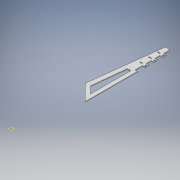
# Autodesk Inventor part: bok
Saved by Autodesk Inventor 2017 (Build 210142000, 142)
## iProperties
Created: 2019-10-27
Part Number: bok
Material: Ogólny
Document SubType Name: Modeling
Designer: patry
Density: 1 g/cm^3
Appearance: Domyślna
Author: patry
Autodesk Inventor part; units mm, degrees
ref_plane "YZ Plane" through (0, 0, 0) normal (1, 0, 0) x (0, 1, 0)
ref_plane "XZ Plane" through (0, 0, 0) normal (0, 1, 0) x (-1, 0, 0)
ref_plane "XY Plane" through (0, 0, 0) normal (0, 0, 1) x (1, 0, 0)
sketch "Szkic1" plane through (0, 0, 0) normal (0, 0, 1) x (1, 0, 0)
  line L0 (176.3308, 486.6406) -> (176.3308, 940.0878) construction
  line L1 (146.3308, 1046.0878) -> (146.3308, 531.0878) construction
  line L2 (246.3308, 494.0715) -> (246.3308, 1046.1041) construction
  line L3 (-96.6896, 915.5533) -> (106.9406, 915.5533) construction
  line L4 (106.9406, 482.7854) -> (106.9406, 1180.5533)
  line L5 (106.9406, 482.7854) -> (-19.1, 609.3854)
  line L6 (50.6014, 1180.5533) -> (-19.1, 609.3854)
  line L7 (19.8894, 612.8224) -> (76.2561, 1146.5389)
  line L8 (76.2561, 1146.5389) -> (76.2561, 556.2056)
  line L9 (43.2451, 833.9694) -> (8.8194, 838.1705) construction
  line L10 (76.2561, 556.2056) -> (54.9566, 535.0002) construction
  line L11 (76.2561, 613.2072) -> (106.9406, 613.2072) construction
  line L12 (76.2561, 556.2056) -> (19.8894, 612.8224)
  line L13 (14.654, 575.0721) -> (120.72, 469.0061) construction
  line L14 (10.3406, 579.3854) -> (14.654, 575.0721) construction
  line L15 (-19.1, 622) -> (-19.1, 0) construction
  line L16 (-8.2, 622) -> (-16.1, 622) construction
  line L17 (-6.6931, 622) -> (-1.5069, 622) construction
  line L18 (-19.1, 622) -> (-16.1, 622) construction
  line L19 (7.9, 622) -> (0, 622) construction
  line L20 (10.9, 621.8118) -> (36.4266, 596.2853) construction
  line L21 (36.4266, 596.2853) -> (142.1601, 489.8877) construction
  line L22 (48.0033, 879.023) -> (76.2561, 879.023)
  line L23 (91.9406, 1180.5533) -> (424.3104, 1180.5533) construction
  line L24 (106.9406, 915.5533) -> (383.3104, 915.5533) construction
  line L25 (91.9406, 1180.5533) -> (50.6014, 1180.5533)
  line L26 (106.9406, 1180.5533) -> (50.6014, 1180.5533)
  point P0 (0, 0)
  dimension "d0" = 30
  dimension "d1" = 100
  constraints: 54 end point, 14 point on line, 6 perpendicular, 4 horizontal, 3 vertical, 1 parallel
  measures "d0" distance between parallel lines of L0 L1
  measures "d1" distance between parallel lines of L1 L2
ref_plane "Płaszczyzna konstrukcyjna1" through (0, 0, 5) normal (0, 0, 1) x (1, 0, 0)
extrude "Wyciągnięcie proste4" add sketch "Szkic1" along normal blind 5 contours L5 L6 L25 L26 L4 | L7 L8 L22
sketch "Szkic3" plane through (0, 0, 0) normal (0, 0, -1) x (-1, 0, 0)
  line L0 (-48.0033, 879.023) -> (-19.8894, 612.8224) projected
  line L1 (-19.8894, 612.8224) -> (-76.2561, 556.2056) projected
  line L2 (-76.2561, 556.2056) -> (-76.2561, 879.023) projected
  line L3 (-76.2561, 879.023) -> (-48.0033, 879.023) projected
  line L4 (-106.9406, 1180.5533) -> (-106.9406, 482.7854) projected
  line L5 (-106.9406, 482.7854) -> (19.1, 609.3854) projected
  line L6 (19.1, 609.3854) -> (-50.6014, 1180.5533) projected
  line L7 (-50.6014, 1180.5533) -> (-106.9406, 1180.5533) construction
  line L8 (-106.9406, 482.7854) -> (-106.9406, 1180.5533) projected
  line L9 (-106.9406, 1060.5533) -> (-86.9406, 1060.5533)
  line L10 (-86.9406, 1060.5533) -> (-86.9406, 1100.5533)
  line L11 (-86.9406, 1100.5533) -> (-106.9406, 1100.5533)
  line L12 (-106.9406, 1100.5533) -> (-106.9406, 1060.5533)
  line L13 (-106.9406, 1130.5533) -> (-86.9406, 1130.5533)
  line L14 (-86.9406, 1130.5533) -> (-86.9406, 1180.5533)
  line L15 (-86.9406, 1180.5533) -> (-106.9406, 1180.5533)
  line L16 (-106.9406, 1180.5533) -> (-106.9406, 1130.5533)
  line L17 (-106.9406, 1030.5533) -> (-86.9406, 1030.5533)
  line L18 (-86.9406, 1030.5533) -> (-86.9406, 990.5533)
  line L19 (-86.9406, 990.5533) -> (-106.9406, 990.5533)
  line L20 (-106.9406, 990.5533) -> (-106.9406, 1030.5533)
  line L21 (-226, 915.5533) -> (53, 915.5533) construction
  line L22 (-86.9406, 990.5533) -> (-106.9406, 990.5533)
  line L23 (-106.9406, 990.5533) -> (-106.9406, 960.5533)
  line L24 (-106.9406, 960.5533) -> (-86.9406, 960.5533)
  line L25 (-86.9406, 960.5533) -> (-106.9406, 960.5533)
  line L26 (-106.9406, 960.5533) -> (-106.9406, 900.5533)
  line L27 (-106.9406, 900.5533) -> (-86.9406, 900.5533)
  line L28 (-86.9406, 900.5533) -> (-86.9406, 960.5533)
  line L29 (-101.9406, 968.0533) -> (-95.9406, 968.0533)
  line L30 (-95.9406, 968.0533) -> (-95.9406, 983.0533)
  line L31 (-95.9406, 983.0533) -> (-101.9406, 983.0533)
  line L32 (-101.9406, 983.0533) -> (-101.9406, 968.0533)
  line L33 (-101.9406, 1038.0533) -> (-95.9406, 1038.0533)
  line L34 (-95.9406, 1038.0533) -> (-95.9406, 1053.0533)
  line L35 (-95.9406, 1053.0533) -> (-101.9406, 1053.0533)
  line L36 (-101.9406, 1053.0533) -> (-101.9406, 1038.0533)
  line L37 (-101.9406, 1108.0533) -> (-95.9406, 1108.0533)
  line L38 (-95.9406, 1108.0533) -> (-95.9406, 1123.0533)
  line L39 (-95.9406, 1123.0533) -> (-101.9406, 1123.0533)
  line L40 (-101.9406, 1123.0533) -> (-101.9406, 1108.0533)
  point P0 (0, 0)
  dimension "d28" = 265
  dimension "d30" = 30
  dimension "d31" = 30
  dimension "d32" = 40
  dimension "d33" = 40
  dimension "d34" = 30
  dimension "d38" = 20
  dimension "d39" = 6
  dimension "d40" = 15
  dimension "d41" = 6
  dimension "d42" = 15
  dimension "d43" = 6
  dimension "d44" = 15
  dimension "d45" = 7.5
  dimension "d46" = 7.5
  dimension "d47" = 7.5
  dimension "d48" = 5
  dimension "d49" = 5
  dimension "d64" = 50
  constraints: 64 end point, 15 parallel, 9 horizontal, 9 point on line, 8 perpendicular, 1 collinear
  measures "d28" distance between parallel lines of L7 L21
  measures "d30" distance between parallel lines of L13 L11
  measures "d31" distance between parallel lines of L17 L9
  measures "d32" distance between parallel lines of L11 L9
  measures "d33" distance between parallel lines of L17 L19
  measures "d34" distance between parallel lines of L19 L24
  measures "d38" distance between parallel lines of L8 L14
  measures "d39" distance of L35.end L34.end
  measures "d40" distance of L34.end L33.end
  measures "d41" distance of L39.end L38.end
  measures "d42" distance of L38.end L37.end
  measures "d43" distance of L30.end L31.end
  measures "d44" distance of L29.end L30.end
  measures "d45" distance between parallel lines of L24 L29
  measures "d46" distance from line of L33.end L17
  measures "d47" distance from line of L37.end L11
  measures "d48" distance between parallel lines of L4 L32
  measures "d49" distance between parallel lines of L4 L36
  measures "d64" distance between parallel lines of L7 L13
extrude "Wyciągnięcie proste5" cut sketch "Szkic3" against normal blind 5 contours L15 L14 L13 L4 | L11 L10 L9 L4 | L17 L18 L19 L4 | L24 L28 L27 L4 | L32 L31 L30 L29 | L36 L35 L34 L33 | L40 L39 L38 L37
fillet "Zaokrąglenie1" radius 2 12 edges at (101.9406, 968.0533, 2.5) (95.9406, 968.0533, 2.5) (95.9406, 983.0533, 2.5) (101.9406, 983.0533, 2.5) (101.9406, 1053.0533, 2.5) (101.9406, 1038.0533, 2.5) (95.9406, 1038.0533, 2.5) (95.9406, 1053.0533, 2.5) (95.9406, 1123.0533, 2.5) (95.9406, 1108.0533, 2.5) (101.9406, 1108.0533, 2.5) (101.9406, 1123.0533, 2.5)
sketch "Szkic4" plane through (0, 0, 5) normal (0, 0, 1) x (1, 0, 0)
  line L0 (19.8894, 612.8224) -> (48.0033, 879.023) projected
  line L1 (48.0033, 879.023) -> (76.2561, 879.023) projected
  line L2 (76.2561, 879.023) -> (76.2561, 556.2056) projected
  line L3 (76.2561, 556.2056) -> (19.8894, 612.8224) projected
  line L4 (95.9406, 1110.0533) -> (95.9406, 1121.0533) projected
  arc A0 (97.9406, 1123.0533) -> (95.9406, 1121.0533) centre (97.9406, 1121.0533) ccw projected
  line L5 (97.9406, 1123.0533) -> (99.9406, 1123.0533) projected
  arc A1 (101.9406, 1121.0533) -> (99.9406, 1123.0533) centre (99.9406, 1121.0533) ccw projected
  line L6 (101.9406, 1121.0533) -> (101.9406, 1110.0533) projected
  arc A2 (99.9406, 1108.0533) -> (101.9406, 1110.0533) centre (99.9406, 1110.0533) ccw projected
  line L7 (99.9406, 1108.0533) -> (97.9406, 1108.0533) projected
  arc A3 (95.9406, 1110.0533) -> (97.9406, 1108.0533) centre (97.9406, 1110.0533) ccw projected
  line L8 (95.9406, 970.0533) -> (95.9406, 981.0533) projected
  arc A4 (97.9406, 983.0533) -> (95.9406, 981.0533) centre (97.9406, 981.0533) ccw projected
  line L9 (97.9406, 983.0533) -> (99.9406, 983.0533) projected
  arc A5 (101.9406, 981.0533) -> (99.9406, 983.0533) centre (99.9406, 981.0533) ccw projected
  line L10 (101.9406, 981.0533) -> (101.9406, 970.0533) projected
  arc A6 (99.9406, 968.0533) -> (101.9406, 970.0533) centre (99.9406, 970.0533) ccw projected
  line L11 (99.9406, 968.0533) -> (97.9406, 968.0533) projected
  arc A7 (95.9406, 970.0533) -> (97.9406, 968.0533) centre (97.9406, 970.0533) ccw projected
  line L12 (95.9406, 1040.0533) -> (95.9406, 1051.0533) projected
  arc A8 (97.9406, 1053.0533) -> (95.9406, 1051.0533) centre (97.9406, 1051.0533) ccw projected
  line L13 (97.9406, 1053.0533) -> (99.9406, 1053.0533) projected
  arc A9 (101.9406, 1051.0533) -> (99.9406, 1053.0533) centre (99.9406, 1051.0533) ccw projected
  line L14 (101.9406, 1051.0533) -> (101.9406, 1040.0533) projected
  arc A10 (99.9406, 1038.0533) -> (101.9406, 1040.0533) centre (99.9406, 1040.0533) ccw projected
  line L15 (99.9406, 1038.0533) -> (97.9406, 1038.0533) projected
  arc A11 (95.9406, 1040.0533) -> (97.9406, 1038.0533) centre (97.9406, 1040.0533) ccw projected
  line L16 (106.9406, 990.5533) -> (86.9406, 990.5533) projected
  line L17 (86.9406, 990.5533) -> (86.9406, 1030.5533) projected
  line L18 (86.9406, 1030.5533) -> (106.9406, 1030.5533) projected
  line L19 (106.9406, 1030.5533) -> (106.9406, 1060.5533) projected
  line L20 (106.9406, 1060.5533) -> (86.9406, 1060.5533) projected
  line L21 (86.9406, 1060.5533) -> (86.9406, 1100.5533) projected
  line L22 (86.9406, 1100.5533) -> (106.9406, 1100.5533) projected
  line L23 (106.9406, 1100.5533) -> (106.9406, 1130.5533) projected
  line L24 (106.9406, 1130.5533) -> (86.9406, 1130.5533) projected
  line L25 (86.9406, 1130.5533) -> (86.9406, 1180.5533) projected
  line L26 (86.9406, 1180.5533) -> (50.6014, 1180.5533) projected
  line L27 (50.6014, 1180.5533) -> (-19.1, 609.3854) projected
  line L28 (-19.1, 609.3854) -> (106.9406, 482.7854) projected
  line L29 (106.9406, 482.7854) -> (106.9406, 900.5533) projected
  line L30 (106.9406, 900.5533) -> (86.9406, 900.5533) projected
  line L31 (86.9406, 900.5533) -> (86.9406, 960.5533) projected
  line L32 (86.9406, 960.5533) -> (106.9406, 960.5533) projected
  line L33 (106.9406, 960.5533) -> (106.9406, 990.5533) projected
  line L34 (51.9406, 972.5533) -> (71.9406, 972.5533)
  line L35 (71.9406, 972.5533) -> (71.9406, 978.5533)
  line L36 (71.9406, 978.5533) -> (51.9406, 978.5533)
  line L37 (51.9406, 978.5533) -> (51.9406, 972.5533)
  line L38 (51.9406, 1042.5533) -> (71.9406, 1042.5533)
  line L39 (71.9406, 1042.5533) -> (71.9406, 1048.5533)
  line L40 (71.9406, 1048.5533) -> (51.9406, 1048.5533)
  line L41 (51.9406, 1048.5533) -> (51.9406, 1042.5533)
  line L42 (51.9406, 1112.5533) -> (71.9406, 1112.5533)
  line L43 (71.9406, 1112.5533) -> (71.9406, 1118.5533)
  line L44 (71.9406, 1118.5533) -> (51.9406, 1118.5533)
  line L45 (51.9406, 1118.5533) -> (51.9406, 1112.5533)
  point P0 (0, 0)
  dimension "d51" = 20
  dimension "d52" = 6
  dimension "d53" = 20
  dimension "d54" = 6
  dimension "d55" = 20
  dimension "d56" = 6
  dimension "d57" = 64
  dimension "d58" = 64
  dimension "d59" = 12
  dimension "d60" = 15
  constraints: 24 end point, 6 parallel, 3 horizontal, 3 perpendicular, 2 vertical alignment
  measures "d51" distance of L35.end L36.end
  measures "d52" distance of L34.end L35.end
  measures "d53" distance of L39.end L40.end
  measures "d54" distance of L38.end L39.end
  measures "d55" distance of L43.end L44.end
  measures "d56" distance of L42.end L43.end
  measures "d57" distance between parallel lines of L38 L36
  measures "d58" distance between parallel lines of L40 L42
  measures "d59" distance between parallel lines of L32 L34
  measures "d60" distance between parallel lines of L17 L35
extrude "Wyciągnięcie proste6" cut sketch "Szkic4" against normal blind 5 contours L37 L36 L35 L34 | L41 L40 L39 L38 | L45 L44 L43 L42
fillet "Zaokrąglenie2" radius 2 12 edges at (51.9406, 972.5533, 2.5) (71.9406, 972.5533, 2.5) (71.9406, 978.5533, 2.5) (51.9406, 978.5533, 2.5) (51.9406, 1048.5533, 2.5) (51.9406, 1042.5533, 2.5) (71.9406, 1042.5533, 2.5) (71.9406, 1048.5533, 2.5) (71.9406, 1118.5533, 2.5) (51.9406, 1118.5533, 2.5) (71.9406, 1112.5533, 2.5) (51.9406, 1112.5533, 2.5)
equation "\"d30\" = d34"
equation "\"d31\" = d34"
equation "\"d32\" = d33"
equation "\"d39\" = d43"
equation "\"d40\" = d44"
equation "\"d41\" = d43"
equation "\"d42\" = d40"
equation "\"d46\" = d45"
equation "\"d47\" = d46"
equation "\"d49\" = d48"
equation "\"d53\" = d51"
equation "\"d55\" = d51"
equation "\"d58\" = d57"
